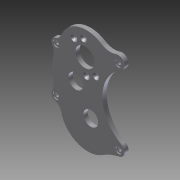
# Autodesk Inventor part: connected plate
Saved by Autodesk Inventor 2012 (Build 160160000, 160)
## iProperties
Created: 2012-01-30
Part Number: connected plate
Material: Default
Document SubType Name: Modeling
Designer: Antonella Wilby
Density: 1 g/cm^3
Mass: 59.3603 g
Surface Area: 248.356 cm^2
Volume: 59.3603 cm^3
Author: Antonella Wilby
Autodesk Inventor part; units mm, degrees
ref_plane "YZ Plane" through (0, 0, 0) normal (1, 0, 0) x (0, 1, 0)
ref_plane "XZ Plane" through (0, 0, 0) normal (0, 1, 0) x (-1, 0, 0)
ref_plane "XY Plane" through (0, 0, 0) normal (0, 0, 1) x (1, 0, 0)
sketch "Sketch1" plane through (0, 0, 0) normal (0, 0, 1) x (1, 0, 0)
  circle A0 centre (0, 0) radius 53.975 construction
  circle A1 centre (-95.7467, 0) radius 11.1125
  circle A2 centre (-73.1257, -37.5239) radius 11.1125
  line L0 (-195.0218, 0) -> (95.4745, 0) projected
  line L1 (0, -186.751) -> (0, 135.7508) projected
  circle A3 centre (-82.0671, 38.2685) radius 14.2875
  arc A4 (-27.1037, 48.5034) -> (-27.1037, -48.5034) centre (0, 0) ccw
  arc A5 (-27.1037, 48.5034) -> (-34.976, 65.7804) centre (-31.75, 56.8183) ccw
  circle A6 centre (-95.7467, 0) radius 33.02 construction
  arc A7 (-57.3305, 68.3238) -> (-118.1642, 48.9464) centre (-79.7457, 33.5145) ccw
  arc A8 (-57.3305, 68.3238) -> (-34.976, 65.7804) centre (-43.5788, 89.6792) ccw
  arc A9 (-29.7745, -66.1362) -> (-27.1037, -48.5034) centre (-31.75, -56.8183) ccw
  arc A10 (-118.11, -50.8) -> (-55.2575, -76.6338) centre (-77.6901, -41.8358) ccw
  arc A11 (-29.7745, -66.1362) -> (-55.2575, -76.6338) centre (-13.9704, -140.6793) ccw
  circle A12 centre (-82.0671, 38.2685) radius 33.02 construction
  circle A13 centre (-73.1257, -37.5239) radius 39.37 construction
  circle A14 centre (-95.7467, 0) radius 10.16 construction
  circle A15 centre (0, 0) radius 16.51 construction
  circle A16 centre (-73.1257, -37.5239) radius 16.51 construction
  line L2 (0, 0) -> (-82.0671, 38.2685) construction
  circle A17 centre (-125.73, 34.29) radius 6.35 construction
  circle A18 centre (-125.73, -34.29) radius 6.35 construction
  line L3 (0, 0) -> (-34.976, 65.7804) construction
  line L4 (0, 0) -> (-57.3305, 68.3238) construction
  arc A19 (-127.2489, 41.2704) -> (-132.0785, 31.0144) centre (-125.73, 34.29) ccw
  arc A20 (-130.3268, 13.3001) -> (-130.3268, -13.3001) centre (-83.9357, 0) ccw
  arc A21 (-130.3268, 13.3001) -> (-132.0785, 31.0144) centre (-153.5223, 19.9501) ccw
  arc A22 (-132.0785, -31.0144) -> (-127.4503, -41.2235) centre (-125.73, -34.29) ccw
  arc A23 (-132.0785, -31.0144) -> (-130.3268, -13.3001) centre (-153.5223, -19.9501) ccw
  arc A24 (-118.11, -50.8) -> (-127.4503, -41.2235) centre (-130.5087, -53.5498) ccw
  arc A25 (-127.2489, 41.2704) -> (-118.1642, 48.9464) centre (-129.949, 53.6801) ccw
  line L5 (-118.1642, 48.9464) -> (0, 48.9464) construction
  line L6 (-118.11, -50.8) -> (0, -50.8) construction
  dimension "d0" = 107.95
  dimension "d9" = 22.225
  dimension "d38" = 28.575
  dimension "d63" = 1.5875
  dimension "d66" = 9.525
  dimension "d77" = 31.75
  dimension "d93" = 66.04
  dimension "d95" = 25.4
  dimension "d106" = 66.04
  dimension "d107" = 78.74
  dimension "d108" = 20.32
  dimension "d110" = 33.02
  dimension "d116" = 43.815
  dimension "d117" = 40.64
  dimension "d118" = 33.02
  dimension "d119" = 22.225
  dimension "d120" = 65
  dimension "d121" = 90.551
  dimension "d125" = 12.7
  dimension "d126" = 12.7
  dimension "d128" = 28
  dimension "d129" = 40
  dimension "d130" = 34.29
  dimension "d131" = 125.73
  dimension "d133" = 34.29
  dimension "d134" = 125.73
  dimension "d141" = 14.2875
  dimension "d144" = 14.2875
  dimension "d145" = 11.811
  dimension "d146" = 24.13
  dimension "d147" = 24.13
  dimension "d150" = 48.26
  dimension "d151" = 12.7
  dimension "d152" = 12.7
  dimension "d153" = 41.402
  dimension "d155" = 76.2
  dimension "d156" = 31.75
  dimension "d157" = 9.525
  dimension "d158" = 118.11
  dimension "d159" = 50.8
  constraints: 30 point on circle, 26 centre point, 14 tangent, 11 coincident, 10 end point, 2 horizontal alignment, 2 perpendicular, 2 point on line, 1 equal radius
  measures "d0" diameter of A0
  measures "d9" diameter of A1
  measures "d38" diameter of A3
  measures "d63" radial gap between concentric circles of A4 A0
  measures "d66" radius of A5
  measures "d77" distance from line of L1 A5.centre
  measures "d93" diameter of A6
  measures "d95" radius of A8
  measures "d106" diameter of A12
  measures "d107" diameter of A13
  measures "d108" diameter of A14
  measures "d110" diameter of A15
  measures "d116" distance of A2.centre A1.centre
  measures "d117" distance of A3.centre A6.centre
  measures "d118" diameter of A16
  measures "d119" diameter of A2
  measures "d120" angle of L1 L2
  measures "d121" distance of L2.start L2.end
  measures "d125" diameter of A17
  measures "d126" diameter of A18
  measures "d128" angle of L1 L3
  measures "d129" angle of L1 L4
  measures "d130" distance from line of A17.centre L0
  measures "d131" distance from line of L1 A17.centre
  measures "d133" distance from line of L0 A18.centre
  measures "d134" distance from line of L1 A18.centre
  measures "d141" diameter of A19
  measures "d144" diameter of A22
  measures "d145" distance of A20.centre A6.centre
  measures "d146" radius of A21
  measures "d147" radius of A23
  measures "d150" radius of A20
  measures "d151" radius of A24
  measures "d152" radius of A25
  measures "d153" radius of A7
  measures "d155" radius of A11
  measures "d156" distance from line of L1 A9.centre
  measures "d157" radius of A9
  measures "d158" distance of L6.start L6.end
  measures "d159" distance between parallel lines of L0 L6
extrude "Base" add sketch "Sketch1" along normal mid plane 6.35 contours L0 A4 A9 A11 A10 A24 A22 A23 A20 A1 | A1 L0 A20 A21 A19 A25 A7 A8 A5 A4
sketch "Sketch4" plane through (0, 0, 3.175) normal (0, 0, 1) x (1, 0, 0)
  circle A0 centre (-82.0671, 38.2685) radius 14.2875 projected
  line L0 (-98.6536, 55.0567) -> (-84.2659, 61.7657) construction
  line L1 (-79.8682, 14.7713) -> (-65.4806, 21.4803) construction
  line L2 (-155.0035, 0) -> (-0.0953, 0) projected
  line L3 (0, -114.8687) -> (0, 106.5474) projected
  line L4 (-72.6744, 18.1258) -> (-91.4598, 58.4112) construction
  point P0 (-82.0671, 38.2685)
  dimension "d122" = 15.875
  dimension "d123" = 44.45
  dimension "d124" = 25
  constraints: 6 end point, 3 midpoint, 2 parallel, 1 coincident, 1 perpendicular
  measures "d122" distance of L0.end L0.start
  measures "d123" distance of L0.start L1.start
  measures "d124" angle of L3 L4
hole "Encoder Mount Holes" at (-98.6536, 55.0567, 3.175) at (-84.2659, 61.7657, 3.175) at (-79.8682, 14.7713, 3.175) at (-65.4806, 21.4803, 3.175) direction (0, 0, -1) diameter 5.1054 end through all countersink diameter 9.779 countersink angle 82 clearance for "Flat Head Machine Screw (82)" size "#10" standard "Ansi Unified Screw Threads"
sketch "Sketch5" plane through (0, 0, 3.175) normal (0, 0, 1) x (1, 0, 0)
  arc A0 (-27.1037, 48.5034) -> (-27.1037, -48.5034) centre (0, 0) ccw projected
  line L0 (0, 0) -> (-31.75, 54.9926) construction
  line L1 (-159.4485, 0) -> (26.5747, 0) construction
  line L2 (0, -114.8687) -> (0, 106.5474) construction
  line L3 (-30.9294, -58.1697) -> (0, 0) construction
  dimension "d64" = 30
  dimension "d65" = 63.5
  dimension "d100" = 65.8812
  dimension "d102" = 62
  constraints: 4 end point
  measures "d64" angle of L2 L0
  measures "d65" distance of L0.start L0.end
  measures "d100" distance of L3.start L0.start
  measures "d102" angle of L1 L3
hole "Standoff holes to motor plate" at (-31.75, 54.9926, 3.175) at (-30.9294, -58.1697, 3.175) direction (0, 0, -1) diameter 5.1054 end through all counterbore diameter 9.779 counterbore depth 1.5875 clearance for "Flat Head Machine Screw (82)" size "#10" standard "Ansi Unified Screw Threads"
sketch "Sketch7" plane through (0, 0, 3.175) normal (0, 0, 1) x (1, 0, 0)
  arc A0 (-127.2489, 41.2704) -> (-132.0785, 31.0144) centre (-125.73, 34.29) ccw projected
  arc A1 (-132.0785, -31.0144) -> (-127.4503, -41.2235) centre (-125.73, -34.29) ccw projected
  constraints: 2 coincident
hole "Standoff holes to front plate" at (-125.73, 34.29, 3.175) at (-125.73, -34.29, 3.175) direction (0, 0, -1) diameter 5.1054 end through all counterbore diameter 9.779 counterbore depth 1.5875 clearance for "Flat Head Machine Screw (82)" size "#10" standard "Ansi Unified Screw Threads"
body "Solid1"
